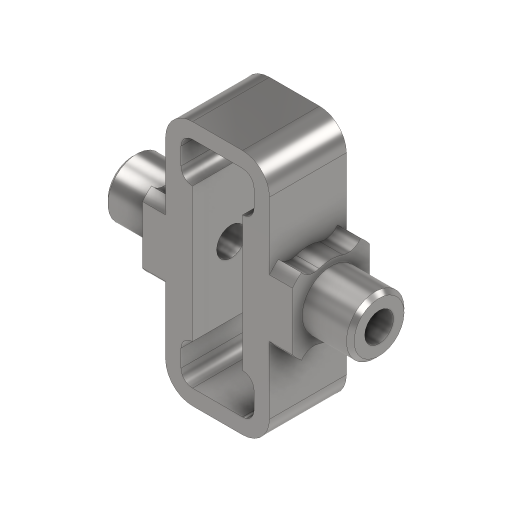
# Autodesk Inventor part: Part036.Connecting cross
Saved by Autodesk Inventor 2023.2 (Build 272271030, 271C)
## iProperties
Created: 2023-11-16
Part Number: Part036.Connecting cross
Material: Steel, Carbon
Document SubType Name: Modeling
Designer: User
Mass: 1459.85 g
Surface Area: 447.665 cm^2
Volume: 185.968 cm^3
Density: 7.85 g/cm^3
Appearance: Semi-Polished
Author: User
Autodesk Inventor part; units mm, degrees
ref_plane "YZ Plane" through (0, 0, 0) normal (1, 0, 0) x (0, 1, 0)
ref_plane "XZ Plane" through (0, 0, 0) normal (0, 1, 0) x (-1, 0, 0)
ref_plane "XY Plane" through (0, 0, 0) normal (0, 0, 1) x (1, 0, 0)
sketch "Sketch1" plane through (0, 0, 0) normal (0, 0, 1) x (1, 0, 0)
  line L0 (-27, -64) -> (27, -64)
  line L1 (27, -64) -> (27, 64)
  line L2 (27, 64) -> (-27, 64)
  line L3 (-27, 64) -> (-27, -64)
  line L4 (-27, -64) -> (27, 64) construction
  line L5 (27, -64) -> (-27, 64) construction
  line L6 (-13, 56) -> (13, 56)
  line L7 (19, 50) -> (19, 41)
  line L8 (13, 35) -> (13, 35)
  line L9 (-19, 41) -> (-19, 50)
  arc A0 (-13, 56) -> (-19, 50) centre (-13, 50) ccw
  arc A1 (19, 50) -> (13, 56) centre (13, 50) ccw
  arc A2 (13, 35) -> (19, 41) centre (13, 41) ccw
  arc A3 (-19, 41) -> (-13, 35) centre (-13, 41) ccw
  line L10 (-37.8, 0) -> (37.8, 0) construction
  line L11 (-27, 64) -> (27, -64) construction
  line L12 (-13, -56) -> (13, -56)
  line L13 (19, -50) -> (19, -41)
  line L14 (13, -35) -> (13, -35)
  line L15 (-19, -41) -> (-19, -50)
  arc A4 (-19, -50) -> (-13, -56) centre (-13, -50) ccw
  arc A5 (13, -56) -> (19, -50) centre (13, -50) ccw
  arc A6 (19, -41) -> (13, -35) centre (13, -41) ccw
  arc A7 (-13, -35) -> (-19, -41) centre (-13, -41) ccw
  line L16 (-13, 35) -> (-13, -35)
  line L17 (13, 35) -> (13, -35)
  line L18 (0, -89.6) -> (0, 89.6) construction
  line L19 (-13, 35) -> (-13, 35)
  line L20 (13, 35) -> (-13, 35) construction
  line L21 (-13, -35) -> (-13, -35)
  line L22 (13, -35) -> (-13, -35) construction
  point P0 (0, 0)
  point P1 (0, 56)
  point P2 (0, 0)
  point P3 (13, 35)
  point P4 (13, -35)
  point P5 (-13, -35)
  point P6 (-13, 35)
  dimension "d0" = 54
  dimension "d1" = 128
  dimension "d2" = 38
  dimension "d3" = 6
  dimension "d4" = 35
  dimension "d5" = 8
  dimension "d6" = 26
  constraints: 42 end point, 16 point on circle, 12 symmetric about line, 12 tangent, 8 centre point, 8 perpendicular, 6 parallel, 4 midpoint, 3 equal radius, 2 horizontal, 1 vertical alignment, 5 other
  measures "d0" distance of L2.end L1.end
  measures "d1" distance of L1.end L0.end
  measures "d2" distance between parallel lines of L7 L9
  measures "d3" radius of A0
  measures "d4" distance from line of point (0, 0) L8
  measures "d5" distance between parallel lines of L6 L2
  measures "d6" distance between parallel lines of L17 L16
extrude "Extrusion1" add sketch "Sketch1" along normal mid plane 40
fillet "Fillet1" radius 14 4 edges at (27, -64, 0) (-27, -64, 0) (-27, 64, 0) (27, 64, 0)
sketch "Sketch2" plane through (27, -50, 20) normal (1, 0, 0) x (0, 0, -1)
  line L0 (0, 0) -> (0, 100) projected
  line L1 (40, 100) -> (40, 0) projected
  arc A0 (0, 35) -> (4.6393, 30.2757) centre (20, 50) ccw
  arc A1 (0, 65) -> (0, 35) centre (20, 50) ccw construction
  arc A2 (40, 65) -> (35.3607, 69.7243) centre (20, 50) ccw
  arc A3 (40, 35) -> (40, 65) centre (20, 50) ccw construction
  line L2 (0, 65) -> (0, 35)
  line L3 (0, 15) -> (0, 85) projected
  line L4 (40, 85) -> (40, 15) projected
  line L5 (40, 65) -> (40, 35)
  circle A4 centre (20, 50) radius 18 construction
  line L6 (11.1075, 74.432) -> (20, 50) construction
  line L7 (28.8925, 74.432) -> (20, 50) construction
  line L8 (20, -39.6) -> (20, 139.6) construction
  line L9 (11.1075, 74.432) -> (28.8925, 74.432) construction
  arc A5 (26.1564, 66.9145) -> (13.8436, 66.9145) centre (20, 50) ccw
  arc A6 (4.6393, 69.7243) -> (13.8436, 66.9145) centre (11.1075, 74.432) ccw
  arc A7 (19.1075, 74.432) -> (19.0885, 74.9834) centre (11.1075, 74.432) ccw construction
  arc A8 (20.9115, 74.9834) -> (20.8925, 74.432) centre (28.8925, 74.432) ccw construction
  arc A9 (26.1564, 66.9145) -> (35.3607, 69.7243) centre (28.8925, 74.432) ccw
  arc A10 (4.6393, 69.7243) -> (0, 65) centre (20, 50) ccw
  arc A11 (35.3607, 69.7243) -> (4.6393, 69.7243) centre (20, 50) ccw construction
  line L10 (55, 50) -> (-15, 50) construction
  circle A12 centre (20, 50) radius 18 construction
  line L11 (11.1075, 25.568) -> (20, 50) construction
  line L12 (28.8925, 25.568) -> (20, 50) construction
  line L13 (20, 139.6) -> (20, -39.6) construction
  arc A13 (13.8436, 33.0855) -> (26.1564, 33.0855) centre (20, 50) ccw
  arc A14 (13.8436, 33.0855) -> (4.6393, 30.2757) centre (11.1075, 25.568) ccw
  arc A15 (35.3607, 30.2757) -> (26.1564, 33.0855) centre (28.8925, 25.568) ccw
  arc A16 (4.6393, 30.2757) -> (35.3607, 30.2757) centre (20, 50) ccw construction
  arc A17 (35.3607, 30.2757) -> (40, 35) centre (20, 50) ccw
  point P0 (20, 74.432)
  dimension "d10" = 50
  dimension "d11" = 36
  dimension "d15" = 40
  constraints: 42 point on circle, 18 centre point, 16 end point, 12 point on line, 8 symmetric about line, 4 coincident, 2 collinear, 1 midpoint, 4 other
  measures "d10" diameter of A0
  measures "d11" diameter of A4
  measures "d15" angle of L7 L6
extrude "Extrusion2" add sketch "Sketch2" along normal blind 12
sketch "Sketch3" plane through (39, -50, 20) normal (1, 0, 0) x (0, 0, -1)
  arc A0 (40, 65) -> (35.3607, 69.7243) centre (20, 50) ccw projected
  circle A1 centre (20, 50) radius 15
  dimension "d18" = 30
  constraints: 1 centre point, 1 coincident
  measures "d18" diameter of A1
extrude "Extrusion3" add sketch "Sketch3" along normal blind 25
chamfer "Chamfer1" distance 2 angle 45 1 edges at (64, 0, 15)
mirror "Mirror1" about plane through (0, 0, 0) normal (1, 0, 0) of "Extrusion2", "Extrusion3", "Chamfer1"
sketch "Sketch4" plane through (-64, 0, 0) normal (-1, 0, 0) x (0, 0, 1)
  circle A0 centre (0, 0) radius 13 projected
  point P0 (0, 0)
  constraints: 1 coincident
hole "Hole1" at (-64, 0, 0) direction (1, 0, 0) diameter 15 end through all
body "Solid1"
